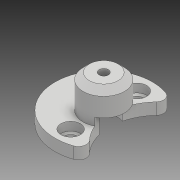
# Autodesk Inventor part: gearbox_axle3_support
Saved by Autodesk Inventor 2017 SP1 (Build 210196100, 196)
## iProperties
Created: 2018-01-26
Part Number: gearbox_axle3_support
Material: Generic
Document SubType Name: Modeling
Designer: JT
Density: 1 g/cm^3
Appearance: Default
Author: JT
Autodesk Inventor part; units mm, degrees
ref_plane "YZ Plane" through (0, 0, 0) normal (1, 0, 0) x (0, 1, 0)
ref_plane "XZ Plane" through (0, 0, 0) normal (0, 1, 0) x (-1, 0, 0)
ref_plane "XY Plane" through (0, 0, 0) normal (0, 0, 1) x (1, 0, 0)
sketch "Sketch1" plane through (0, 0, 0) normal (0, 0, 1) x (1, 0, 0)
  circle A0 centre (0, 0) radius 6.25
  dimension "d0" = 12.5
  constraints: 1 centre point, 1 coincident
  measures "d0" diameter of A0
extrude "Extrusion1" add sketch "Sketch1" along normal blind 1.5
sketch "axles" plane through (0, 0, 0) normal (0, 0, 1) x (1, 0, 0)
  point P0 (0, 0)
  point P1 (7, 0)
  point P2 (0.3, 0)
  dimension "d3" = 7
  dimension "d4" = 6.7
  constraints: 2 horizontal alignment
  measures "d3" distance of point (7, 0) point (0, 0)
  measures "d4" distance of point (7, 0) point (0.3, 0)
sketch "Sketch4" plane through (0, 0, 1.5) normal (0, 0, 1) x (1, 0, 0)
  circle A0 centre (0, 0) radius 2.65
  dimension "d8" = 5.3
  constraints: 1 centre point, 1 coincident
  measures "d8" diameter of A0
extrude "Extrusion3" add sketch "Sketch4" along normal blind 4.2
chamfer "Chamfer1" distance 0.8 angle 45 1 edges at (-2.65, 0, 5.7)
sketch "Sketch5" plane through (0, 0, 0) normal (0, 0, 1) x (1, 0, 0)
  circle A0 centre (0.3, 0) radius 1.6
  point P0 (0, 0)
  dimension "d14" = 3.2
  constraints: 1 centre point, 1 coincident
  measures "d14" diameter of A0
extrude "motor shaft" cut sketch "Sketch5" along normal blind 2.5
sketch "Sketch6" plane through (0, 0, 0) normal (0, 0, -1) x (-1, 0, 0)
  circle A0 centre (-7, 0) radius 6.25
  point P0 (0, 0)
  dimension "d17" = 12.5
  constraints: 1 centre point, 1 coincident
  measures "d17" diameter of A0
extrude "Extrusion5" cut sketch "Sketch6" against normal blind 2.5
sketch "Sketch8" plane through (0, 0, 5.7) normal (0, 0, 1) x (1, 0, 0)
  point P0 (0, 0)
  point P1 (0, 0)
  constraints: 1 coincident
hole "Hole1" at (0, 0, 5.7) direction (0, 0, -1) diameter 1.2 end through all
fillet "Fillet1" radius 1 2 edges at (3.5, 5.1781, 0.75) (3.5, -5.1781, 0.75)
sketch "Sketch9" plane through (0, 0, 1.5) normal (0, 0, 1) x (1, 0, 0)
  line L0 (0, -4.25) -> (0, 4.25) construction
  point P0 (0, 0)
  point P1 (0, 0)
  dimension "d28" = 8.5
  constraints: 3 coincident, 2 end point, 1 midpoint, 1 vertical
  measures "d28" distance of L0.start L0.end
hole "Hole2" at (0, -4.25, 1.5) at (0, 4.25, 1.5) direction (0, 0, -1) diameter 1.5 end through all counterbore diameter 2.5 counterbore depth 1.1
equation "\"axle_dist_2_3__3_4\" = 7"
equation "\"axle_dist_1_2\" = 6.7"
body "Solid1"
